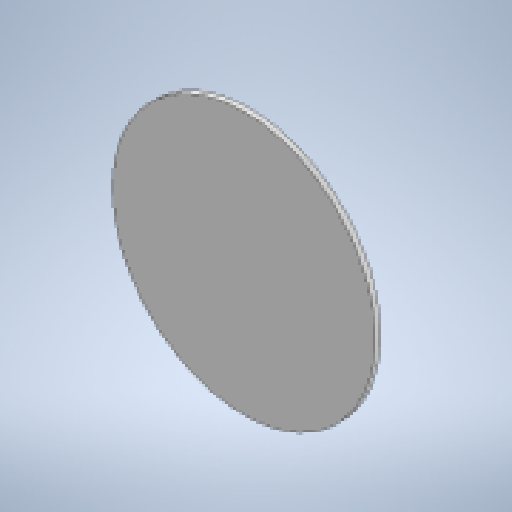
# Autodesk Inventor part: Base_Plato
Saved by Autodesk Inventor 2024 (Build 280153000, 153)
## iProperties
Created: 2024-07-17
Part Number: Base_Plato
Material: Genérico
Document SubType Name: Modeling
Designer: sergi
Density: 1 g/cm^3
Appearance: Valor por defecto
Author: sergi
Autodesk Inventor part; units mm, degrees
ref_plane "YZ Plane" through (0, 0, 0) normal (1, 0, 0) x (0, 1, 0)
ref_plane "XZ Plane" through (0, 0, 0) normal (0, 1, 0) x (-1, 0, 0)
ref_plane "XY Plane" through (0, 0, 0) normal (0, 0, 1) x (1, 0, 0)
sketch "Boceto1" plane through (0, 0, 0) normal (0, 0, 1) x (1, 0, 0)
  circle A0 centre (-24.75, 100) radius 51.4081 projected
  circle A1 centre (-24.75, 100) radius 70
  point P0 (0, 0)
  dimension "d0" = 140
  constraints: 1 centre point, 1 coincident
  measures "d0" diameter of A1
extrude "Extrusión1" add sketch "Boceto1" along normal blind 3 contours A0 | A1
sketch "Boceto2" plane through (-24.75, 100, 0) normal (0, 0, -1) x (-1, 0, 0)
  circle A0 centre (0, 0) radius 6.4
  point P0 (-24.75, -100)
  dimension "d3" = 12.8
  constraints: 1 centre point
  measures "d3" diameter of A0
extrude "Extrusión2" add sketch "Boceto2" along normal blind 10
sketch "Boceto3" plane through (-24.75, 100, -10) normal (0, 0, -1) x (-1, 0, 0)
  circle A0 centre (0, 0) radius 6.4 projected
  point P0 (-24.75, -100)
  constraints: 1 coincident
hole "Agujero1" at (-24.75, 100, -10) direction (0, 0, 1) diameter 5.6 depth 4
fillet "Empalme1" radius 3 1 edges at (-18.35, 100, 0)
